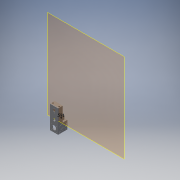
# Autodesk Inventor part: Xendmotorside
Saved by Autodesk Inventor 2016 (Build 200138000, 138)
## iProperties
Created: 2016-05-27
Part Number: Xendmotorside
Material: Generic
Document SubType Name: Modeling
Designer: Scott
Density: 1 g/cm^3
Appearance: Default
Author: Scott
Autodesk Inventor part; units mm, degrees
ref_plane "YZ Plane" through (0, 0, 0) normal (1, 0, 0) x (0, 1, 0)
ref_plane "XZ Plane" through (0, 0, 0) normal (0, 1, 0) x (-1, 0, 0)
ref_plane "XY Plane" through (0, 0, 0) normal (0, 0, 1) x (1, 0, 0)
ref_plane "Work Plane1" through (0, 0, 0) normal (0, 0, 1) x (1, 0, 0)
sketch "Sketch1" plane through (0, 0, 0) normal (0, 0, 1) x (1, 0, 0)
  circle A0 centre (0, 0) radius 6.35 projected
  circle A1 centre (0.5752, -49.1016) radius 4 projected
  line L0 (-12.7, -22.86) -> (12.7, -22.86)
  line L1 (12.7, -22.86) -> (12.7, 22.86)
  line L2 (12.7, 22.86) -> (-12.7, 22.86)
  line L3 (-12.7, 22.86) -> (-12.7, -22.86)
  line L4 (-12.7, -22.86) -> (12.7, 22.86) construction
  line L5 (12.7, -22.86) -> (-12.7, 22.86) construction
  line L6 (12.7, 22.86) -> (-12.7, 22.86)
  line L7 (-12.7, 22.86) -> (-12.7, -66.04)
  line L8 (-12.7, -66.04) -> (12.7, -66.04)
  line L9 (12.7, -66.04) -> (12.7, 22.86)
  point P0 (0, 0)
  dimension "d0" = 25.4
  dimension "d1" = 45.72
  dimension "d2" = 88.9
  constraints: 20 end point, 4 parallel, 2 horizontal, 2 midpoint, 2 perpendicular
  measures "d0" distance of L2.end L1.end
  measures "d1" distance of L1.end L0.end
  measures "d2" distance of L7.end L6.end
extrude "Extrusion1" add sketch "Sketch1" along normal blind 2.54
sketch "Sketch2" plane through (0, 0, 2.54) normal (0, 0, 1) x (1, 0, 0)
  circle A0 centre (0, 0) radius 6.35 projected
  circle A1 centre (0.5752, -49.1016) radius 4 projected
  line L0 (12.7, 22.86) -> (-12.7, 22.86) projected
  line L1 (-12.7, 22.86) -> (-12.7, -66.04) projected
  line L2 (-12.7, -66.04) -> (12.7, -66.04) projected
  line L3 (12.7, -66.04) -> (12.7, 22.86) projected
  circle A2 centre (0, 0) radius 7.62
  line L4 (0, 0) -> (0, -12.7)
  circle A3 centre (0, -12.7) radius 2.54
  line L5 (0, 0) -> (0, 12.7)
  circle A4 centre (0, 12.7) radius 2.54
  circle A5 centre (0.5752, -49.1016) radius 4 projected
  circle A6 centre (0.5752, -49.1016) radius 5
  point P0 (0, 0)
  dimension "d5" = 15.24
  dimension "d6" = 12.7
  dimension "d7" = 5.08
  dimension "d8" = 12.7
  dimension "d9" = 5.08
  dimension "d10" = 10
  constraints: 4 centre point, 4 coincident, 4 end point, 2 vertical
  measures "d5" diameter of A2
  measures "d6" distance of L4.start L4.end
  measures "d7" diameter of A3
  measures "d8" distance of L4.start L5.end
  measures "d9" diameter of A4
  measures "d10" diameter of A6
extrude "Extrusion2" cut sketch "Sketch2" against normal blind 2.54 contours A0 L4 L5 | A0 L5 A2 L4 | L5 L4 A0 | A0 L4 A2 L5 | A3 | A4 | A6
sketch "Sketch3" plane through (0, 0, 0) normal (0, 0, -1) x (-1, 0, 0)
  circle A0 centre (0, 0) radius 7.62 projected
  circle A1 centre (0, 12.7) radius 2.54 projected
  circle A2 centre (0, -12.7) radius 2.54 projected
  circle A3 centre (-0.5752, -49.1016) radius 5 projected
  line L0 (-12.7, 22.86) -> (12.7, 22.86) projected
  line L1 (-12.7, -66.04) -> (-12.7, 22.86) projected
  line L2 (12.7, -66.04) -> (-12.7, -66.04) projected
  line L3 (12.7, 22.86) -> (12.7, -66.04) projected
  line L4 (10.16, 19.05) -> (-10.16, 19.05)
  line L5 (-10.16, 19.05) -> (-10.16, -19.05)
  line L6 (-10.16, -19.05) -> (10.16, -19.05)
  line L7 (10.16, -19.05) -> (10.16, 19.05)
  circle A4 centre (0, 0) radius 7.62 projected
  line L8 (10.16, 19.05) -> (-10.16, -19.05) construction
  line L9 (-10.16, 19.05) -> (10.16, -19.05) construction
  point P0 (0, 0)
  dimension "d13" = 20.32
  dimension "d14" = 38.1
  constraints: 12 end point, 2 midpoint, 2 parallel, 1 horizontal, 1 perpendicular
  measures "d13" distance of L6.end L5.end
  measures "d14" distance of L5.end L4.end
extrude "Extrusion3" add sketch "Sketch3" along normal blind 25.4 contours L0 L3 L2 L1
sketch "Sketch4" plane through (0, 0, 2.54) normal (0, 0, 1) x (1, 0, 0)
  line L0 (-12.7, -66.04) -> (12.7, -66.04) projected
  line L1 (0, -66.04) -> (0, -90.8431)
  line L2 (24.81, -115.6589) -> (-24.81, -115.6589)
  line L3 (-24.81, -115.6589) -> (-24.81, -66.0273)
  line L4 (-24.81, -66.0273) -> (24.81, -66.0273)
  line L5 (24.81, -66.0273) -> (24.81, -115.6589)
  line L6 (24.81, -115.6589) -> (-24.81, -66.0273) construction
  line L7 (-24.81, -115.6589) -> (24.81, -66.0273) construction
  circle A0 centre (0, -90.8431) radius 12.5
  line L8 (0, -90.8431) -> (-15.5, -90.8431)
  line L9 (-15.5, -90.8431) -> (-15.5, -75.3431)
  circle A1 centre (-15.5, -75.3431) radius 2
  circle A2 centre (-15.5, -106.3467) radius 2
  circle A3 centre (15.5, -106.3467) radius 2
  circle A4 centre (15.5, -75.3395) radius 2
  point P0 (0, 0)
  dimension "d17" = 24.8031
  dimension "d18" = 49.62
  dimension "d19" = 49.6316
  dimension "d20" = 25
  dimension "d21" = 15.5
  dimension "d22" = 15.5
  dimension "d23" = 4
  dimension "d24" = 4
  dimension "d25" = 4
  dimension "d26" = 4
  constraints: 18 end point, 5 centre point, 3 midpoint, 3 point on line, 2 coincident, 2 horizontal, 2 parallel, 2 vertical, 1 perpendicular
  measures "d17" distance of L1.start L1.end
  measures "d18" distance of L3.end L4.end
  measures "d19" distance of L2.end L3.end
  measures "d20" diameter of A0
  measures "d21" distance of L8.start L8.end
  measures "d22" distance of L8.end L9.end
  measures "d23" diameter of A1
  measures "d24" diameter of A2
  measures "d25" diameter of A3
  measures "d26" diameter of A4
extrude "Extrusion4" add sketch "Sketch4" against normal blind 5.08
sketch "Sketch5" plane through (0, 0, -2.54) normal (0, 0, -1) x (-1, 0, 0)
  circle A0 centre (0, -90.8431) radius 12.5 projected
  circle A1 centre (-15.5, -75.3395) radius 2 projected
  circle A2 centre (-15.5, -106.3467) radius 2 projected
  circle A3 centre (15.5, -106.3467) radius 2 projected
  circle A4 centre (15.5, -75.3431) radius 2 projected
  line L0 (-12.7, -66.0273) -> (-12.7, 22.86) projected
  line L1 (-12.7, 22.86) -> (12.7, 22.86) projected
  line L2 (12.7, 22.86) -> (12.7, -66.0273) projected
  line L3 (24.81, -66.0273) -> (12.7, -66.0273) projected
  line L4 (24.81, -115.6589) -> (24.81, -66.0273) projected
  line L5 (-24.81, -115.6589) -> (24.81, -115.6589) projected
  line L6 (-24.81, -66.0273) -> (-24.81, -115.6589) projected
  line L7 (-12.7, -66.0273) -> (-24.81, -66.0273) projected
  circle A5 centre (0, 0) radius 7.62 projected
  circle A6 centre (0, 12.7) radius 2.54 projected
  circle A7 centre (0, -12.7) radius 2.54 projected
  circle A8 centre (-0.5752, -49.1016) radius 5 projected
  line L8 (24.81, -66.0273) -> (12.7, -66.0273) projected
  line L9 (-24.81, -115.6589) -> (24.81, -115.6589)
  line L10 (24.81, -115.6589) -> (24.81, -66.0273)
  line L11 (24.81, -66.0273) -> (-24.81, -66.0273)
  line L12 (-24.81, -66.0273) -> (-24.81, -115.6589)
  line L13 (-24.81, -115.6589) -> (24.81, -66.0273) construction
  line L14 (24.81, -115.6589) -> (-24.81, -66.0273) construction
  line L15 (-22, -112.8431) -> (22, -112.8431)
  line L16 (22, -112.8431) -> (22, -68.8431)
  line L17 (22, -68.8431) -> (-22, -68.8431)
  line L18 (-22, -68.8431) -> (-22, -112.8431)
  line L19 (-22, -112.8431) -> (22, -68.8431) construction
  line L20 (22, -112.8431) -> (-22, -68.8431) construction
  point P0 (0, 0)
  dimension "d29" = 44
  dimension "d30" = 44
  constraints: 24 end point, 4 midpoint, 4 parallel, 2 horizontal, 2 perpendicular
  measures "d29" distance of L17.end L16.end
  measures "d30" distance of L16.end L15.end
extrude "Extrusion5" add sketch "Sketch5" along normal blind 50.8 contours L11 L3 L4 L5 L6 L7
sketch "Sketch6" plane through (0, 0, -53.34) normal (0, 0, -1) x (-1, 0, 0)
  line L0 (22, -68.8431) -> (22, -112.8431) projected
  line L1 (22, -112.8431) -> (50.6459, -112.8431)
  line L2 (50.6459, -112.8431) -> (50.6459, -68.8431)
  line L3 (50.6459, -68.8431) -> (22, -68.8431)
  line L4 (22, -68.8431) -> (22, -112.8431)
  point P0 (0, 0)
  constraints: 8 end point, 2 parallel, 1 horizontal, 1 perpendicular
extrude "Extrusion6" cut sketch "Sketch6" against normal blind 50.8
chamfer "Chamfer1" distance 44.45 angle 45 1 edges at (-24.81, -114.251, -53.34)
sketch "Sketch7" plane through (12.7, -66.0273, 2.54) normal (0, 1, 0) x (1, 0, 0)
  line L0 (-25.4, 27.94) -> (-25.4, 0) projected
  line L1 (0, 27.94) -> (-25.4, 27.94) projected
  line L2 (0, 0) -> (0, 27.94) projected
  line L3 (0, 0) -> (12.11, 0) projected
  line L4 (12.11, 0) -> (12.11, 55.88) projected
  line L5 (-37.51, 55.88) -> (12.11, 55.88) projected
  line L6 (-37.51, 0) -> (-37.51, 55.88) projected
  line L7 (-37.51, 0) -> (-25.4, 0) projected
  line L8 (6.055, 0) -> (6.055, 12.7)
  circle A0 centre (6.055, 12.7) radius 4
  circle A1 centre (-31.455, 12.7) radius 4
  line L9 (0, 27.94) -> (12.11, 27.94)
  line L10 (12.11, 0) -> (12.11, 55.88) projected
  line L11 (-25.4, 27.94) -> (-37.51, 27.94)
  line L12 (-37.51, 55.88) -> (-37.51, 5.08) projected
  point P0 (-12.7, 2.54)
  dimension "d38" = 12.7
  dimension "d39" = 8
  dimension "d40" = 8
  constraints: 6 end point, 2 centre point, 2 midpoint, 2 point on line, 1 coincident, 1 vertical
  measures "d38" distance of L8.start L8.end
  measures "d39" diameter of A0
  measures "d40" diameter of A1
extrude "Extrusion7" add sketch "Sketch7" along normal up to surface (88.8873 mm away) contours L0 L7 L6 L11 | L9 L4 L3 L2
sketch "Sketch8" plane through (0, 0, -25.4) normal (0, 0, -1) x (-1, 0, 0)
  line L0 (24.81, -66.0273) -> (-24.81, -66.0273) projected
  line L1 (24.81, -66.0273) -> (24.81, 22.86) projected
  line L2 (24.81, 22.86) -> (-24.81, 22.86) projected
  line L3 (-24.81, -66.0273) -> (-24.81, 22.86) projected
  line L4 (10.16, 19.05) -> (10.16, -19.05) projected
  line L5 (10.16, -19.05) -> (-10.16, -19.05) projected
  line L6 (-10.16, -19.05) -> (-10.16, 19.05) projected
  line L7 (-10.16, 19.05) -> (10.16, 19.05) projected
  circle A0 centre (-0.5752, -49.1016) radius 5 projected
  circle A1 centre (-0.5752, -49.1016) radius 12.7
  point P0 (0, 0)
  dimension "d43" = 25.4
  constraints: 1 centre point, 1 coincident
  measures "d43" diameter of A1
extrude "Extrusion8" add sketch "Sketch8" along normal blind 12.7 contours A1
sketch "Sketch9" plane through (0.5752, -49.1016, -38.1) normal (0, 0, -1) x (-1, 0, 0)
  circle A0 centre (0, 0) radius 12.7 projected
  line L0 (25.3852, -16.9257) -> (-24.2348, -16.9257) projected
  line L1 (25.3852, -16.9257) -> (25.3852, 71.9616) projected
  line L2 (25.3852, 71.9616) -> (-24.2348, 71.9616) projected
  line L3 (-24.2348, -16.9257) -> (-24.2348, 71.9616) projected
  line L4 (10.7352, 68.1516) -> (10.7352, 30.0516) projected
  line L5 (10.7352, 30.0516) -> (-9.5848, 30.0516) projected
  line L6 (-9.5848, 30.0516) -> (-9.5848, 68.1516) projected
  line L7 (-9.5848, 68.1516) -> (10.7352, 68.1516) projected
  line L8 (-12.7, 0) -> (-12.7, -16.9257)
  line L9 (25.3852, -16.9257) -> (-24.2348, -16.9257) projected
  circle A1 centre (0, 0) radius 12.7 projected
  line L10 (12.7, 0) -> (12.7, -16.9257)
  line L11 (12.7, -16.9257) -> (-12.7, -16.9257)
  point P0 (0.5752, 49.1016)
  constraints: 6 end point, 2 perpendicular, 2 point on circle, 2 point on line, 1 collinear, 1 horizontal alignment, 1 vertical, 1 other
extrude "Extrusion9" add sketch "Sketch9" against normal up to surface (12.7 mm away) contours L10 L0 L8 A0
sketch "Sketch10" plane through (0, 0, -38.1) normal (0, 0, -1) x (-1, 0, 0)
  circle A0 centre (-0.5752, -49.1016) radius 5 projected
  circle A1 centre (-0.5752, -49.1016) radius 7.5
  point P0 (0, 0)
  dimension "d48" = 15
  constraints: 1 centre point, 1 coincident
  measures "d48" diameter of A1
sketch "Sketch11" plane through (0, 0, 2.54) normal (0, 0, 1) x (1, 0, 0)
  circle A0 centre (0.5752, -49.1016) radius 5 projected
  circle A1 centre (0.5752, -49.1016) radius 7.5
  point P0 (0, 0)
  dimension "d49" = 15
  constraints: 1 centre point, 1 coincident
  measures "d49" diameter of A1
extrude "Extrusion10" cut sketch "Sketch11" against normal blind 24
sketch "Sketch12" plane through (0, 0, -38.1) normal (0, 0, -1) x (-1, 0, 0)
  circle A0 centre (-0.5752, -49.1016) radius 5 projected
  arc A1 (12.1248, -49.1016) -> (-13.2752, -49.1016) centre (-0.5752, -49.1016) ccw projected
  line L0 (-13.2752, -49.1016) -> (-13.2752, -66.0273) projected
  line L1 (12.1248, -66.0273) -> (-13.2752, -66.0273) projected
  line L2 (12.1248, -66.0273) -> (12.1248, -49.1016) projected
  point P0 (0, 0)
extrude "Extrusion11" add sketch "Sketch12" along normal blind 8.89
sketch "Sketch13" plane through (0, 0, -46.99) normal (0, 0, -1) x (-1, 0, 0)
  circle A0 centre (-0.5752, -49.1016) radius 5 projected
  arc A1 (12.1248, -49.1016) -> (-13.2752, -49.1016) centre (-0.5752, -49.1016) ccw projected
  line L0 (-13.2752, -49.1016) -> (-13.2752, -66.0273) projected
  line L1 (12.1248, -66.0273) -> (-13.2752, -66.0273) projected
  line L2 (12.1248, -66.0273) -> (12.1248, -49.1016) projected
  circle A2 centre (-0.5752, -49.1016) radius 7.5
  point P0 (0, 0)
  dimension "d54" = 15
  constraints: 1 centre point, 1 coincident
  measures "d54" diameter of A2
extrude "Extrusion12" cut sketch "Sketch13" against normal blind 24 contours A2
sketch "Sketch14" plane through (24.81, -115.6589, 2.54) normal (1, 0, 0) x (0, 0, -1)
  spline S0 degree 2 poles (6.6012, 5.0914) (10.3495, 6.6696) (13.0128, 10.9605) knots 0 0 0 1 1 1
  spline S1 degree 2 poles (13.0128, 10.9605) (14.6897, 14.0677) (14.6897, 14.6102) knots 0 0 0 1 1 1
  line L0 (14.6897, 14.6102) -> (14.2952, 14.6102)
  spline S2 degree 2 poles (14.2952, 14.6102) (13.0128, 14.6102) (8.8206, 7.0642) knots 0 0 0 1 1 1
  line L1 (8.8206, 7.0642) -> (8.722, 7.0642)
  line L2 (8.722, 7.0642) -> (8.722, 7.3108)
  spline S3 degree 2 poles (8.722, 7.3108) (11.3359, 12.7854) (11.3359, 16.583) knots 0 0 0 1 1 1
  spline S4 degree 2 poles (11.3359, 16.583) (11.3359, 18.0133) (9.1165, 23.192) knots 0 0 0 1 1 1
  spline S5 degree 2 poles (9.1165, 23.192) (8.574, 25.3621) (8.574, 26.743) knots 0 0 0 1 1 1
  line L3 (8.574, 26.743) -> (8.574, 28.272)
  spline S6 degree 2 poles (8.574, 28.272) (8.574, 35.67) (12.6183, 45.8793) knots 0 0 0 1 1 1
  line L4 (12.6183, 45.8793) -> (12.8649, 46.9151)
  line L5 (12.8649, 46.9151) -> (13.1608, 46.9151)
  line L6 (13.1608, 46.9151) -> (13.1608, 45.0902)
  spline S7 degree 2 poles (13.1608, 45.0902) (13.2594, 42.0817) (13.654, 42.0817) knots 0 0 0 1 1 1
  spline S8 degree 2 poles (13.654, 42.0817) (17.4517, 43.4133) (20.0656, 43.4133) knots 0 0 0 1 1 1
  spline S9 degree 2 poles (20.0656, 43.4133) (24.9484, 43.4133) (30.9654, 38.7279) knots 0 0 0 1 1 1
  spline S10 degree 2 poles (30.9654, 38.7279) (37.0812, 31.6257) (38.9554, 22.3042) knots 0 0 0 1 1 1
  spline S11 degree 2 poles (38.9554, 22.3042) (39.4486, 19.4929) (39.4486, 14.7582) knots 0 0 0 1 1 1
  line L7 (39.4486, 14.7582) -> (39.4486, 13.969)
  spline S12 degree 2 poles (39.4486, 13.969) (41.8159, 7.5574) (46.8466, 5.0914) knots 0 0 0 1 1 1
  spline S13 degree 2 poles (46.8466, 5.0914) (47.2412, 5.0914) (47.2412, 4.8448) knots 0 0 0 1 1 1
  line L8 (47.2412, 4.8448) -> (46.452, 4.5982)
  line L9 (46.452, 4.5982) -> (46.3534, 4.5982)
  spline S14 degree 2 poles (46.3534, 4.5982) (44.4299, 4.5982) (39.5472, 9.7768) knots 0 0 0 1 1 1
  line L10 (39.5472, 9.7768) -> (39.5472, 9.6782)
  line L11 (39.5472, 9.6782) -> (39.6952, 7.5574)
  line L12 (39.6952, 7.5574) -> (39.6952, 7.3108)
  line L13 (39.6952, 7.3108) -> (39.4486, 7.3108)
  spline S15 degree 2 poles (39.4486, 7.3108) (38.1169, 12.7854) (35.6509, 14.6102) knots 0 0 0 1 1 1
  spline S16 degree 2 poles (35.6509, 14.6102) (35.6509, 14.8568) (34.3686, 14.8568) knots 0 0 0 1 1 1
  line L14 (34.3686, 14.8568) -> (31.3107, 14.8568)
  line L15 (31.3107, 14.8568) -> (31.3107, 11.7496)
  spline S17 degree 2 poles (31.3107, 11.7496) (31.3107, 11.3057) (33.2342, 10.9605) knots 0 0 0 1 1 1
  line L16 (33.2342, 10.9605) -> (33.2342, 10.7139)
  line L17 (33.2342, 10.7139) -> (26.0334, 10.7139)
  line L18 (26.0334, 10.7139) -> (26.0334, 10.9605)
  spline S18 degree 2 poles (26.0334, 10.9605) (26.6746, 10.9605) (27.3157, 12.1442) knots 0 0 0 1 1 1
  line L19 (27.3157, 12.1442) -> (27.3157, 14.8568)
  line L20 (27.3157, 14.8568) -> (21.5946, 14.8568)
  line L21 (21.5946, 14.8568) -> (21.348, 15.1527)
  line L22 (21.348, 15.1527) -> (21.5946, 16.2871)
  spline S19 degree 2 poles (21.5946, 16.2871) (21.2493, 17.8654) (20.0656, 17.8654) knots 0 0 0 1 1 1
  spline S20 degree 2 poles (20.0656, 17.8654) (18.3887, 17.8654) (17.6983, 14.3636) knots 0 0 0 1 1 1
  spline S21 degree 2 poles (17.6983, 14.3636) (16.12, 11.6017) (10.9414, 6.5217) knots 0 0 0 1 1 1
  spline S22 degree 2 poles (10.9414, 6.5217) (8.5247, 4.7461) (7.5383, 4.7461) knots 0 0 0 1 1 1
  line L23 (7.5383, 4.7461) -> (7.3903, 4.7461)
  spline S23 degree 2 poles (7.3903, 4.7461) (6.6012, 4.8448) (6.6012, 5.0914) knots 0 0 0 1 1 1
  line L24 (17.6983, 20.6273) -> (27.3157, 20.6273)
  spline S24 degree 2 poles (27.3157, 20.6273) (27.3157, 22.4522) (25.0963, 23.0933) knots 0 0 0 1 1 1
  spline S25 degree 2 poles (25.0963, 23.0933) (24.7511, 23.0933) (24.7511, 23.3399) knots 0 0 0 1 1 1
  line L25 (24.7511, 23.3399) -> (24.7511, 23.4879)
  line L26 (24.7511, 23.4879) -> (33.9247, 23.4879)
  spline S26 degree 2 poles (33.9247, 23.4879) (33.7274, 22.9947) (31.7053, 22.3042) knots 0 0 0 1 1 1
  line L27 (31.7053, 22.3042) -> (31.3107, 20.6273)
  line L28 (31.3107, 20.6273) -> (34.6152, 20.6273)
  spline S27 degree 2 poles (34.6152, 20.6273) (34.2206, 23.8331) (33.3328, 26.3485) knots 0 0 0 1 1 1
  spline S28 degree 2 poles (33.3328, 26.3485) (32.2478, 28.9131) (29.9297, 31.2805) knots 0 0 0 1 1 1
  line L29 (29.9297, 31.2805) -> (29.9297, 31.4285)
  line L30 (29.9297, 31.4285) -> (30.5709, 31.4285)
  spline S29 degree 2 poles (30.5709, 31.4285) (32.7903, 31.0832) (36.3414, 22.6988) knots 0 0 0 1 1 1
  line L31 (36.3414, 22.6988) -> (36.9825, 20.6273)
  spline S30 degree 2 poles (36.9825, 20.6273) (37.821, 20.6273) (38.0183, 21.7617) knots 0 0 0 1 1 1
  spline S31 degree 2 poles (38.0183, 21.7617) (35.7495, 30.0968) (30.3243, 33.8945) knots 0 0 0 1 1 1
  spline S32 degree 2 poles (30.3243, 33.8945) (26.132, 37.1496) (20.7068, 37.1496) knots 0 0 0 1 1 1
  spline S33 degree 2 poles (20.7068, 37.1496) (14.2952, 37.1496) (11.4346, 32.0696) knots 0 0 0 1 1 1
  spline S34 degree 2 poles (11.4346, 32.0696) (10.7934, 30.2448) (10.7934, 28.4199) knots 0 0 0 1 1 1
  spline S35 degree 2 poles (10.7934, 28.4199) (10.7934, 22.9947) (13.1608, 21.5151) knots 0 0 0 1 1 1
  spline S36 degree 2 poles (13.1608, 21.5151) (14.5911, 20.6273) (17.6983, 20.6273) knots 0 0 0 1 1 1
  point P0 (2.54, 115.6589)
  point P1 (6.6012, 7.5081)
  constraints: 1 other
extrude "Extrusion13" add sketch "Sketch14" along normal blind 1.27
sketch "Sketch15" plane through (24.81, -115.6589, 2.54) normal (1, 0, 0) x (0, 0, -1)
  spline S0 degree 2 poles (44.1908, 6.1802) (45.1279, 6.5747) (45.7937, 7.6474) knots 0 0 0 1 1 1
  spline S1 degree 2 poles (45.7937, 7.6474) (46.2129, 8.4242) (46.2129, 8.5599) knots 0 0 0 1 1 1
  line L0 (46.2129, 8.5599) -> (46.1143, 8.5599)
  spline S2 degree 2 poles (46.1143, 8.5599) (45.7937, 8.5599) (44.7457, 6.6734) knots 0 0 0 1 1 1
  line L1 (44.7457, 6.6734) -> (44.721, 6.6734)
  line L2 (44.721, 6.6734) -> (44.721, 6.735)
  spline S3 degree 2 poles (44.721, 6.735) (45.3745, 8.1036) (45.3745, 9.0531) knots 0 0 0 1 1 1
  spline S4 degree 2 poles (45.3745, 9.0531) (45.3745, 9.4106) (44.8196, 10.7053) knots 0 0 0 1 1 1
  spline S5 degree 2 poles (44.8196, 10.7053) (44.684, 11.2478) (44.684, 11.5931) knots 0 0 0 1 1 1
  line L3 (44.684, 11.5931) -> (44.684, 11.9753)
  spline S6 degree 2 poles (44.684, 11.9753) (44.684, 13.8248) (45.6951, 16.3771) knots 0 0 0 1 1 1
  line L4 (45.6951, 16.3771) -> (45.7567, 16.6361)
  line L5 (45.7567, 16.6361) -> (45.8307, 16.6361)
  line L6 (45.8307, 16.6361) -> (45.8307, 16.1799)
  spline S7 degree 2 poles (45.8307, 16.1799) (45.8554, 15.4277) (45.954, 15.4277) knots 0 0 0 1 1 1
  spline S8 degree 2 poles (45.954, 15.4277) (46.9034, 15.7606) (47.5569, 15.7606) knots 0 0 0 1 1 1
  spline S9 degree 2 poles (47.5569, 15.7606) (48.7776, 15.7606) (50.2819, 14.5893) knots 0 0 0 1 1 1
  spline S10 degree 2 poles (50.2819, 14.5893) (51.8108, 12.8137) (52.2793, 10.4834) knots 0 0 0 1 1 1
  spline S11 degree 2 poles (52.2793, 10.4834) (52.4026, 9.7805) (52.4026, 8.5969) knots 0 0 0 1 1 1
  line L7 (52.4026, 8.5969) -> (52.4026, 8.3996)
  spline S12 degree 2 poles (52.4026, 8.3996) (52.9945, 6.7967) (54.2522, 6.1802) knots 0 0 0 1 1 1
  spline S13 degree 2 poles (54.2522, 6.1802) (54.3508, 6.1802) (54.3508, 6.1185) knots 0 0 0 1 1 1
  line L8 (54.3508, 6.1185) -> (54.1535, 6.0569)
  line L9 (54.1535, 6.0569) -> (54.1289, 6.0569)
  spline S14 degree 2 poles (54.1289, 6.0569) (53.648, 6.0569) (52.4273, 7.3515) knots 0 0 0 1 1 1
  line L10 (52.4273, 7.3515) -> (52.4273, 7.3269)
  line L11 (52.4273, 7.3269) -> (52.4643, 6.7967)
  line L12 (52.4643, 6.7967) -> (52.4643, 6.735)
  line L13 (52.4643, 6.735) -> (52.4026, 6.735)
  spline S15 degree 2 poles (52.4026, 6.735) (52.0697, 8.1036) (51.4532, 8.5599) knots 0 0 0 1 1 1
  spline S16 degree 2 poles (51.4532, 8.5599) (51.4532, 8.6215) (51.1326, 8.6215) knots 0 0 0 1 1 1
  line L14 (51.1326, 8.6215) -> (50.3682, 8.6215)
  line L15 (50.3682, 8.6215) -> (50.3682, 7.8447)
  spline S17 degree 2 poles (50.3682, 7.8447) (50.3682, 7.7337) (50.8491, 7.6474) knots 0 0 0 1 1 1
  line L16 (50.8491, 7.6474) -> (50.8491, 7.5858)
  line L17 (50.8491, 7.5858) -> (49.0489, 7.5858)
  line L18 (49.0489, 7.5858) -> (49.0489, 7.6474)
  spline S18 degree 2 poles (49.0489, 7.6474) (49.2092, 7.6474) (49.3694, 7.9434) knots 0 0 0 1 1 1
  line L19 (49.3694, 7.9434) -> (49.3694, 8.6215)
  line L20 (49.3694, 8.6215) -> (47.9392, 8.6215)
  line L21 (47.9392, 8.6215) -> (47.8775, 8.6955)
  line L22 (47.8775, 8.6955) -> (47.9392, 8.9791)
  spline S19 degree 2 poles (47.9392, 8.9791) (47.8528, 9.3736) (47.5569, 9.3736) knots 0 0 0 1 1 1
  spline S20 degree 2 poles (47.5569, 9.3736) (47.1377, 9.3736) (46.9651, 8.4982) knots 0 0 0 1 1 1
  spline S21 degree 2 poles (46.9651, 8.4982) (46.5705, 7.8077) (45.2759, 6.5377) knots 0 0 0 1 1 1
  spline S22 degree 2 poles (45.2759, 6.5377) (44.6717, 6.0938) (44.4251, 6.0938) knots 0 0 0 1 1 1
  line L23 (44.4251, 6.0938) -> (44.3881, 6.0938)
  spline S23 degree 2 poles (44.3881, 6.0938) (44.1908, 6.1185) (44.1908, 6.1802) knots 0 0 0 1 1 1
  line L24 (46.9651, 10.0641) -> (49.3694, 10.0641)
  spline S24 degree 2 poles (49.3694, 10.0641) (49.3694, 10.5203) (48.8146, 10.6806) knots 0 0 0 1 1 1
  spline S25 degree 2 poles (48.8146, 10.6806) (48.7283, 10.6806) (48.7283, 10.7423) knots 0 0 0 1 1 1
  line L25 (48.7283, 10.7423) -> (48.7283, 10.7793)
  line L26 (48.7283, 10.7793) -> (51.0217, 10.7793)
  spline S26 degree 2 poles (51.0217, 10.7793) (50.9724, 10.656) (50.4668, 10.4834) knots 0 0 0 1 1 1
  line L27 (50.4668, 10.4834) -> (50.3682, 10.0641)
  line L28 (50.3682, 10.0641) -> (51.1943, 10.0641)
  spline S27 degree 2 poles (51.1943, 10.0641) (51.0957, 10.8656) (50.8737, 11.4944) knots 0 0 0 1 1 1
  spline S28 degree 2 poles (50.8737, 11.4944) (50.6025, 12.1356) (50.0229, 12.7274) knots 0 0 0 1 1 1
  line L29 (50.0229, 12.7274) -> (50.0229, 12.7644)
  line L30 (50.0229, 12.7644) -> (50.1832, 12.7644)
  spline S29 degree 2 poles (50.1832, 12.7644) (50.7381, 12.6781) (51.6259, 10.582) knots 0 0 0 1 1 1
  line L31 (51.6259, 10.582) -> (51.7861, 10.0641)
  spline S30 degree 2 poles (51.7861, 10.0641) (51.9958, 10.0641) (52.0451, 10.3477) knots 0 0 0 1 1 1
  spline S31 degree 2 poles (52.0451, 10.3477) (51.4779, 12.4315) (50.1216, 13.3809) knots 0 0 0 1 1 1
  spline S32 degree 2 poles (50.1216, 13.3809) (49.0735, 14.1947) (47.7172, 14.1947) knots 0 0 0 1 1 1
  spline S33 degree 2 poles (47.7172, 14.1947) (46.1143, 14.1947) (45.3992, 12.9247) knots 0 0 0 1 1 1
  spline S34 degree 2 poles (45.3992, 12.9247) (45.2389, 12.4685) (45.2389, 12.0123) knots 0 0 0 1 1 1
  spline S35 degree 2 poles (45.2389, 12.0123) (45.2389, 10.656) (45.8307, 10.2861) knots 0 0 0 1 1 1
  spline S36 degree 2 poles (45.8307, 10.2861) (46.1883, 10.0641) (46.9651, 10.0641) knots 0 0 0 1 1 1
  line L32 (45.0169, 21.8764) -> (45.806, 21.0502)
  spline S37 degree 2 poles (45.806, 21.0502) (45.806, 21.1859) (45.8677, 21.1859) knots 0 0 0 1 1 1
  line L33 (45.8677, 21.1859) -> (45.9417, 21.1859)
  spline S38 degree 2 poles (45.9417, 21.1859) (45.9787, 21.1859) (46.0526, 20.9393) knots 0 0 0 1 1 1
  line L34 (46.0526, 20.9393) -> (46.1636, 20.7913)
  line L35 (46.1636, 20.7913) -> (46.3856, 20.8283)
  spline S39 degree 2 poles (46.3856, 20.8283) (47.187, 20.8283) (48.2597, 19.8049) knots 0 0 0 1 1 1
  spline S40 degree 2 poles (48.2597, 19.8049) (49.0119, 19.509) (49.1105, 19.509) knots 0 0 0 1 1 1
  line L36 (49.1105, 19.509) -> (51.4409, 19.509)
  spline S41 degree 2 poles (51.4409, 19.509) (51.7122, 19.509) (51.9711, 19.6939) knots 0 0 0 1 1 1
  spline S42 degree 2 poles (51.9711, 19.6939) (52.1067, 19.6939) (52.1067, 19.9405) knots 0 0 0 1 1 1
  line L37 (52.1067, 19.9405) -> (52.3163, 20.3844)
  line L38 (52.3163, 20.3844) -> (52.378, 20.3844)
  line L39 (52.378, 20.3844) -> (52.2793, 19.3117)
  spline S43 degree 2 poles (52.2793, 19.3117) (52.2793, 18.4733) (52.4273, 17.4622) knots 0 0 0 1 1 1
  line L40 (52.4273, 17.4622) -> (52.378, 17.4622)
  spline S44 degree 2 poles (52.378, 17.4622) (52.2177, 18.017) (52.0697, 18.1897) knots 0 0 0 1 1 1
  spline S45 degree 2 poles (52.0697, 18.1897) (52.0697, 18.4239) (51.8355, 18.4239) knots 0 0 0 1 1 1
  spline S46 degree 2 poles (51.8355, 18.4239) (51.5395, 18.5226) (50.0969, 18.6212) knots 0 0 0 1 1 1
  spline S47 degree 2 poles (50.0969, 18.6212) (49.3325, 18.6212) (48.6666, 18.2636) knots 0 0 0 1 1 1
  spline S48 degree 2 poles (48.6666, 18.2636) (46.4595, 17.4129) (46.3609, 17.2526) knots 0 0 0 1 1 1
  line L41 (46.3609, 17.2526) -> (46.3609, 17.1663)
  spline S49 degree 2 poles (46.3609, 17.1663) (46.3609, 16.9443) (46.4842, 16.3155) knots 0 0 0 1 1 1
  line L42 (46.4842, 16.3155) -> (46.4472, 16.3155)
  spline S50 degree 2 poles (46.4472, 16.3155) (46.102, 17.0306) (46.0526, 17.0306) knots 0 0 0 1 1 1
  spline S51 degree 2 poles (46.0526, 17.0306) (45.991, 16.8087) (45.9417, 16.8087) knots 0 0 0 1 1 1
  line L43 (45.9417, 16.8087) -> (45.8677, 16.8087)
  line L44 (45.8677, 16.8087) -> (45.806, 16.858)
  line L45 (45.806, 16.858) -> (45.806, 17.5855)
  line L46 (45.806, 17.5855) -> (45.6088, 18.0664)
  spline S52 degree 2 poles (45.6088, 18.0664) (45.806, 18.1403) (45.806, 18.1897) knots 0 0 0 1 1 1
  line L47 (45.806, 18.1897) -> (45.806, 18.5472)
  line L48 (45.806, 18.5472) -> (45.8677, 18.5966)
  line L49 (45.8677, 18.5966) -> (45.9417, 18.5966)
  spline S53 degree 2 poles (45.9417, 18.5966) (45.991, 18.5966) (46.0526, 18.2636) knots 0 0 0 1 1 1
  spline S54 degree 2 poles (46.0526, 18.2636) (47.1377, 18.7938) (48.0871, 19.398) knots 0 0 0 1 1 1
  spline S55 degree 2 poles (48.0871, 19.398) (48.0871, 19.6323) (47.4336, 19.8049) knots 0 0 0 1 1 1
  spline S56 degree 2 poles (47.4336, 19.8049) (46.7555, 20.1132) (46.5828, 20.1132) knots 0 0 0 1 1 1
  line L50 (46.5828, 20.1132) -> (46.4842, 20.1132)
  spline S57 degree 2 poles (46.4842, 20.1132) (46.3239, 20.0269) (46.3239, 19.7802) knots 0 0 0 1 1 1
  line L51 (46.3239, 19.7802) -> (46.4102, 19.1514)
  line L52 (46.4102, 19.1514) -> (46.1143, 19.62)
  spline S58 degree 2 poles (46.1143, 19.62) (46.0403, 19.62) (46.0033, 19.7186) knots 0 0 0 1 1 1
  spline S59 degree 2 poles (46.0033, 19.7186) (45.806, 19.7186) (45.806, 19.7802) knots 0 0 0 1 1 1
  line L53 (45.806, 19.7802) -> (45.806, 19.9775)
  line L54 (45.806, 19.9775) -> (45.7567, 19.9775)
  line L55 (45.7567, 19.9775) -> (45.7567, 20.0515)
  spline S60 degree 2 poles (45.7567, 20.0515) (45.7567, 20.1748) (45.0169, 21.8517) knots 0 0 0 1 1 1
  line L56 (45.0169, 21.8517) -> (45.0169, 21.8764)
  spline S61 degree 2 poles (45.7937, 26.3029) (45.8307, 26.5371) (45.88, 26.5371) knots 0 0 0 1 1 1
  line L57 (45.88, 26.5371) -> (45.991, 26.5371)
  line L58 (45.991, 26.5371) -> (46.0403, 26.4755)
  line L59 (46.0403, 26.4755) -> (46.0403, 26.2166)
  spline S62 degree 2 poles (46.0403, 26.2166) (46.0403, 25.8343) (46.6198, 25.785) knots 0 0 0 1 1 1
  line L60 (46.6198, 25.785) -> (47.6926, 25.7603)
  line L61 (47.6926, 25.7603) -> (52.452, 25.7603)
  line L62 (52.452, 25.7603) -> (52.5013, 25.711)
  line L63 (52.5013, 25.711) -> (52.5013, 25.6617)
  spline S63 degree 2 poles (52.5013, 25.6617) (52.3657, 25.5014) (51.7368, 25.1315) knots 0 0 0 1 1 1
  line L64 (51.7368, 25.1315) -> (51.7368, 25.0945)
  spline S64 degree 2 poles (51.7368, 25.0945) (52.3163, 24.7493) (52.7479, 24.0588) knots 0 0 0 1 1 1
  line L65 (52.7479, 24.0588) -> (53.1918, 23.5533)
  line L66 (53.1918, 23.5533) -> (53.1918, 23.5286)
  line L67 (53.1918, 23.5286) -> (53.0068, 23.6642)
  line L68 (53.0068, 23.6642) -> (53.3274, 23.134)
  spline S65 degree 2 poles (53.3274, 23.134) (51.8478, 24.5767) (51.2806, 24.7739) knots 0 0 0 1 1 1
  line L69 (51.2806, 24.7739) -> (51.2806, 24.8109)
  line L70 (51.2806, 24.8109) -> (47.7665, 22.4682)
  line L71 (47.7665, 22.4682) -> (50.8367, 22.4436)
  line L72 (50.8367, 22.4436) -> (51.3546, 22.4436)
  spline S66 degree 2 poles (51.3546, 22.4436) (51.7738, 22.4436) (52.0081, 22.6532) knots 0 0 0 1 1 1
  line L73 (52.0081, 22.6532) -> (52.3163, 23.097)
  line L74 (52.3163, 23.097) -> (52.341, 23.097)
  line L75 (52.341, 23.097) -> (52.341, 22.9121)
  line L76 (52.341, 22.9121) -> (52.3903, 22.8381)
  line L77 (52.3903, 22.8381) -> (52.3903, 21.0872)
  line L78 (52.3903, 21.0872) -> (52.341, 21.0379)
  line L79 (52.341, 21.0379) -> (52.2424, 21.0379)
  line L80 (52.2424, 21.0379) -> (52.1807, 21.0872)
  line L81 (52.1807, 21.0872) -> (52.1807, 21.2969)
  spline S67 degree 2 poles (52.1807, 21.2969) (52.1807, 21.7777) (51.3546, 21.7777) knots 0 0 0 1 1 1
  line L82 (51.3546, 21.7777) -> (46.9158, 21.7777)
  spline S68 degree 2 poles (46.9158, 21.7777) (47.0267, 21.4078) (47.9268, 20.4707) knots 0 0 0 1 1 1
  line L83 (47.9268, 20.4707) -> (48.0378, 20.3474)
  line L84 (48.0378, 20.3474) -> (48.0378, 20.3104)
  spline S69 degree 2 poles (48.0378, 20.3104) (47.0637, 21.1242) (46.4102, 21.4325) knots 0 0 0 1 1 1
  line L85 (46.4102, 21.4325) -> (46.4102, 21.4818)
  line L86 (46.4102, 21.4818) -> (46.5212, 21.6174)
  line L87 (46.5212, 21.6174) -> (46.5212, 21.6421)
  spline S70 degree 2 poles (46.5212, 21.6421) (46.0157, 21.2969) (46.0157, 20.742) knots 0 0 0 1 1 1
  line L88 (46.0157, 20.742) -> (45.88, 20.742)
  line L89 (45.88, 20.742) -> (45.8307, 20.7913)
  line L90 (45.8307, 20.7913) -> (45.8307, 22.1476)
  line L91 (45.8307, 22.1476) -> (45.991, 22.3079)
  spline S71 degree 2 poles (45.991, 22.3079) (45.9293, 22.3202) (45.88, 22.4436) knots 0 0 0 1 1 1
  spline S72 degree 2 poles (45.88, 22.4436) (46.1266, 23.3683) (47.3103, 24.6753) knots 0 0 0 1 1 1
  spline S73 degree 2 poles (47.3103, 24.6753) (47.372, 24.6753) (47.8159, 25.0945) knots 0 0 0 1 1 1
  line L92 (47.8159, 25.0945) -> (47.8159, 25.1315)
  line L93 (47.8159, 25.1315) -> (46.6568, 25.1315)
  spline S74 degree 2 poles (46.6568, 25.1315) (46.0403, 25.1315) (46.0403, 24.2437) knots 0 0 0 1 1 1
  line L94 (46.0403, 24.2437) -> (45.991, 24.2437)
  line L95 (45.991, 24.2437) -> (45.991, 24.3301)
  spline S75 degree 2 poles (45.991, 24.3301) (45.991, 24.6753) (45.8554, 24.6753) knots 0 0 0 1 1 1
  line L96 (45.8554, 24.6753) -> (45.8307, 24.7)
  line L97 (45.8307, 24.7) -> (45.8307, 26.1919)
  line L98 (45.8307, 26.1919) -> (45.7937, 26.3029)
  line L99 (47.4213, 23.2573) -> (47.4459, 23.2573)
  line L100 (47.4459, 23.2573) -> (50.1339, 25.0205)
  line L101 (50.1339, 25.0205) -> (50.1339, 25.0452)
  line L102 (50.1339, 25.0452) -> (50.0353, 25.0452)
  spline S76 degree 2 poles (50.0353, 25.0452) (48.8269, 25.0452) (47.6679, 23.6396) knots 0 0 0 1 1 1
  line L103 (47.6679, 23.6396) -> (47.4213, 23.2573)
  line L104 (50.5161, 25.3904) -> (50.6888, 25.3904)
  line L105 (50.6888, 25.3904) -> (50.6888, 25.4151)
  line L106 (50.6888, 25.4151) -> (50.5161, 25.4151)
  line L107 (50.5161, 25.4151) -> (50.5161, 25.3904)
  line L108 (44.9553, 27.4372) -> (44.9553, 27.4619)
  line L109 (44.9553, 27.4619) -> (45.7321, 29.2128)
  line L110 (45.7321, 29.2128) -> (45.7321, 29.3854)
  line L111 (45.7321, 29.3854) -> (45.7567, 29.3854)
  line L112 (45.7567, 29.3854) -> (45.7814, 29.3607)
  line L113 (45.7814, 29.3607) -> (45.806, 29.3607)
  line L114 (45.806, 29.3607) -> (45.7814, 29.9772)
  line L115 (45.7814, 29.9772) -> (45.7814, 31.1116)
  spline S77 degree 2 poles (45.7814, 31.1116) (45.8184, 31.1856) (46.5459, 31.6541) knots 0 0 0 1 1 1
  line L116 (46.5459, 31.6541) -> (46.5705, 31.6541)
  line L117 (46.5705, 31.6541) -> (46.5705, 31.6171)
  spline S78 degree 2 poles (46.5705, 31.6171) (46.2623, 31.1239) (46.2623, 30.976) knots 0 0 0 1 1 1
  spline S79 degree 2 poles (46.2623, 30.976) (46.2623, 30.8034) (46.4595, 30.8034) knots 0 0 0 1 1 1
  line L118 (46.4595, 30.8034) -> (51.8108, 30.828)
  spline S80 degree 2 poles (51.8108, 30.828) (52.0944, 30.828) (52.1684, 31.2842) knots 0 0 0 1 1 1
  line L119 (52.1684, 31.2842) -> (52.23, 31.2842)
  spline S81 degree 2 poles (52.23, 31.2842) (52.341, 31.2472) (52.341, 31.1609) knots 0 0 0 1 1 1
  line L120 (52.341, 31.1609) -> (52.3657, 31.1609)
  line L121 (52.3657, 31.1609) -> (52.9082, 31.6788)
  line L122 (52.9082, 31.6788) -> (52.9082, 31.6541)
  spline S82 degree 2 poles (52.9082, 31.6541) (52.341, 30.9883) (52.341, 30.3718) knots 0 0 0 1 1 1
  line L123 (52.341, 30.3718) -> (52.341, 29.0525)
  line L124 (52.341, 29.0525) -> (52.3163, 29.0155)
  line L125 (52.3163, 29.0155) -> (52.3163, 28.9908)
  spline S83 degree 2 poles (52.3163, 28.9908) (52.156, 28.9908) (52.156, 29.2991) knots 0 0 0 1 1 1
  spline S84 degree 2 poles (52.156, 29.2991) (51.9834, 29.7553) (51.7122, 29.7553) knots 0 0 0 1 1 1
  line L126 (51.7122, 29.7553) -> (50.2202, 29.7553)
  line L127 (50.2202, 29.7553) -> (50.2202, 27.6592)
  line L128 (50.2202, 27.6592) -> (50.2572, 27.6592)
  spline S85 degree 2 poles (50.2572, 27.6592) (51.9218, 28.1031) (51.9218, 28.4606) knots 0 0 0 1 1 1
  line L129 (51.9218, 28.4606) -> (51.9464, 28.4236)
  line L130 (51.9464, 28.4236) -> (52.0081, 28.4236)
  line L131 (52.0081, 28.4236) -> (52.3163, 28.7689)
  line L132 (52.3163, 28.7689) -> (52.341, 28.7689)
  line L133 (52.341, 28.7689) -> (52.341, 28.5963)
  line L134 (52.341, 28.5963) -> (52.3657, 28.4606)
  line L135 (52.3657, 28.4606) -> (52.3903, 28.4606)
  spline S86 degree 2 poles (52.3903, 28.4606) (53.6973, 29.2498) (53.8946, 29.2498) knots 0 0 0 1 1 1
  spline S87 degree 2 poles (53.8946, 29.2498) (52.5383, 27.8811) (52.5383, 27.7702) knots 0 0 0 1 1 1
  line L136 (52.5383, 27.7702) -> (52.452, 27.5729)
  line L137 (52.452, 27.5729) -> (52.6493, 25.97)
  line L138 (52.6493, 25.97) -> (52.5999, 25.97)
  line L139 (52.5999, 25.97) -> (52.3657, 26.6358)
  line L140 (52.3657, 26.6358) -> (52.341, 26.6358)
  line L141 (52.341, 26.6358) -> (52.341, 25.2548)
  line L142 (52.341, 25.2548) -> (52.3163, 25.2548)
  spline S88 degree 2 poles (52.3163, 25.2548) (52.1191, 25.2548) (52.0574, 25.711) knots 0 0 0 1 1 1
  spline S89 degree 2 poles (52.0574, 25.711) (51.6752, 26.1919) (50.8984, 26.7344) knots 0 0 0 1 1 1
  spline S90 degree 2 poles (50.8984, 26.7344) (50.4422, 26.6111) (50.0846, 26.6111) knots 0 0 0 1 1 1
  line L143 (50.0846, 26.6111) -> (49.6777, 26.6111)
  spline S91 degree 2 poles (49.6777, 26.6111) (47.9638, 26.6111) (46.5459, 28.1894) knots 0 0 0 1 1 1
  spline S92 degree 2 poles (46.5459, 28.1894) (46.1513, 28.7936) (46.1513, 28.8799) knots 0 0 0 1 1 1
  line L144 (46.1513, 28.8799) -> (46.1143, 28.8799)
  spline S93 degree 2 poles (46.1143, 28.8799) (46.1143, 28.6086) (45.2142, 27.6838) knots 0 0 0 1 1 1
  spline S94 degree 2 poles (45.2142, 27.6838) (45.0416, 27.4372) (44.9553, 27.4372) knots 0 0 0 1 1 1
  line L145 (49.8257, 27.9181) -> (49.8257, 29.7553)
  line L146 (49.8257, 29.7553) -> (47.9885, 29.7553)
  line L147 (47.9885, 29.7553) -> (47.9885, 29.2498)
  line L148 (47.9885, 29.2498) -> (49.8257, 27.9181)
  line L149 (49.2585, 27.5729) -> (49.653, 27.5729)
  spline S95 degree 2 poles (49.653, 27.5729) (49.6284, 27.6345) (49.2585, 27.8565) knots 0 0 0 1 1 1
  line L150 (49.2585, 27.8565) -> (49.2955, 27.8811)
  line L151 (49.2955, 27.8811) -> (48.1858, 28.6456)
  line L152 (48.1858, 28.6456) -> (48.1611, 28.6456)
  line L153 (48.1611, 28.6456) -> (48.1611, 28.6209)
  spline S96 degree 2 poles (48.1611, 28.6209) (48.6173, 28.0661) (49.2338, 27.8811) knots 0 0 0 1 1 1
  line L154 (49.2338, 27.8811) -> (49.2338, 27.8565)
  line L155 (49.2338, 27.8565) -> (49.1722, 27.8565)
  spline S97 degree 2 poles (49.1722, 27.8565) (47.9392, 28.214) (47.5693, 28.4606) knots 0 0 0 1 1 1
  line L156 (47.5693, 28.4606) -> (47.5323, 28.473)
  line L157 (47.5323, 28.473) -> (47.5323, 28.51)
  line L158 (47.5323, 28.51) -> (47.5693, 29.1018)
  spline S98 degree 2 poles (47.5693, 29.1018) (46.6938, 29.7553) (46.5705, 29.7553) knots 0 0 0 1 1 1
  line L159 (46.5705, 29.7553) -> (46.3239, 29.7553)
  spline S99 degree 2 poles (46.3239, 29.7553) (46.3239, 29.0402) (46.9158, 28.5346) knots 0 0 0 1 1 1
  spline S100 degree 2 poles (46.9158, 28.5346) (48.0255, 27.5729) (49.2585, 27.5729) knots 0 0 0 1 1 1
  spline S101 degree 2 poles (51.8848, 26.5618) (52.156, 26.6111) (52.156, 27.0427) knots 0 0 0 1 1 1
  line L160 (52.156, 27.0427) -> (52.156, 27.092)
  line L161 (52.156, 27.092) -> (52.0081, 27.092)
  spline S102 degree 2 poles (52.0081, 27.092) (51.8108, 27.092) (51.2929, 26.8947) knots 0 0 0 1 1 1
  line L162 (51.2929, 26.8947) -> (51.2929, 26.8701)
  spline S103 degree 2 poles (51.2929, 26.8701) (51.6752, 26.5618) (51.8848, 26.5618) knots 0 0 0 1 1 1
  line L163 (47.5693, 29.5334) -> (47.5939, 29.5334)
  line L164 (47.5939, 29.5334) -> (47.5939, 29.7183)
  line L165 (47.5939, 29.7183) -> (47.5323, 29.7183)
  line L166 (47.5323, 29.7183) -> (47.5323, 29.7553)
  line L167 (47.5323, 29.7553) -> (47.3103, 29.7183)
  line L168 (47.3103, 29.7183) -> (47.5693, 29.5334)
  line L169 (45.6951, 32.9735) -> (45.6951, 33.0351)
  spline S104 degree 2 poles (45.6951, 33.0351) (46.9034, 33.8736) (47.8035, 34.4161) knots 0 0 0 1 1 1
  line L170 (47.8035, 34.4161) -> (47.8035, 34.5024)
  spline S105 degree 2 poles (47.8035, 34.5024) (47.0021, 35.1189) (45.8677, 35.7601) knots 0 0 0 1 1 1
  line L171 (45.8677, 35.7601) -> (45.8307, 35.7847)
  line L172 (45.8307, 35.7847) -> (45.8307, 35.8217)
  line L173 (45.8307, 35.8217) -> (45.8677, 36.6355)
  line L174 (45.8677, 36.6355) -> (45.8307, 37.5602)
  line L175 (45.8307, 37.5602) -> (45.8924, 37.5602)
  line L176 (45.8924, 37.5602) -> (45.8924, 37.5356)
  spline S106 degree 2 poles (45.8924, 37.5356) (45.8924, 37.2273) (46.028, 37.2273) knots 0 0 0 1 1 1
  spline S107 degree 2 poles (46.028, 37.2273) (46.028, 36.6848) (46.5705, 36.6848) knots 0 0 0 1 1 1
  line L177 (46.5705, 36.6848) -> (46.8788, 36.6602)
  line L178 (46.8788, 36.6602) -> (51.3669, 36.6602)
  line L179 (51.3669, 36.6602) -> (51.6259, 36.6355)
  spline S108 degree 2 poles (51.6259, 36.6355) (52.1807, 36.6355) (52.1807, 37.252) knots 0 0 0 1 1 1
  line L180 (52.1807, 37.252) -> (52.3533, 37.252)
  line L181 (52.3533, 37.252) -> (52.3533, 34.9463)
  line L182 (52.3533, 34.9463) -> (52.3287, 34.9463)
  line L183 (52.3287, 34.9463) -> (51.9834, 35.4765)
  spline S109 degree 2 poles (51.9834, 35.4765) (51.5642, 35.6984) (51.4039, 35.6984) knots 0 0 0 1 1 1
  line L184 (51.4039, 35.6984) -> (48.1858, 35.6737)
  line L185 (48.1858, 35.6737) -> (48.0748, 35.6737)
  line L186 (48.0748, 35.6737) -> (48.0748, 35.6491)
  line L187 (48.0748, 35.6491) -> (52.3533, 34.3544)
  line L188 (52.3533, 34.3544) -> (52.3533, 34.2928)
  spline S110 degree 2 poles (52.3533, 34.2928) (52.3533, 34.2188) (50.6641, 33.7379) knots 0 0 0 1 1 1
  line L189 (50.6641, 33.7379) -> (47.261, 32.7269)
  line L190 (47.261, 32.7269) -> (47.261, 32.6899)
  line L191 (47.261, 32.6899) -> (48.42, 32.6405)
  line L192 (48.42, 32.6405) -> (51.1696, 32.6405)
  line L193 (51.1696, 32.6405) -> (51.3423, 32.6899)
  line L194 (51.3423, 32.6899) -> (51.4779, 32.6652)
  spline S111 degree 2 poles (51.4779, 32.6652) (52.1807, 32.6652) (52.1807, 33.2324) knots 0 0 0 1 1 1
  spline S112 degree 2 poles (52.1807, 33.2324) (52.2917, 33.2324) (52.2917, 33.3064) knots 0 0 0 1 1 1
  line L195 (52.2917, 33.3064) -> (52.2917, 33.368)
  line L196 (52.2917, 33.368) -> (52.3533, 33.368)
  line L197 (52.3533, 33.368) -> (52.3533, 33.2817)
  line L198 (52.3533, 33.2817) -> (52.3287, 33.257)
  line L199 (52.3287, 33.257) -> (52.3533, 33.2324)
  line L200 (52.3533, 33.2324) -> (52.3533, 31.4692)
  line L201 (52.3533, 31.4692) -> (52.2917, 31.4692)
  line L202 (52.2917, 31.4692) -> (52.2917, 31.6418)
  spline S113 degree 2 poles (52.2917, 31.6418) (52.2917, 31.6788) (52.156, 31.7158) knots 0 0 0 1 1 1
  spline S114 degree 2 poles (52.156, 31.7158) (52.156, 32.1597) (51.9588, 32.1597) knots 0 0 0 1 1 1
  spline S115 degree 2 poles (51.9588, 32.1597) (51.8108, 32.2213) (51.5642, 32.2213) knots 0 0 0 1 1 1
  line L203 (51.5642, 32.2213) -> (47.2117, 32.1597)
  line L204 (47.2117, 32.1597) -> (46.7061, 32.1843)
  line L205 (46.7061, 32.1843) -> (46.6815, 32.1597)
  line L206 (46.6815, 32.1597) -> (46.6815, 32.024)
  spline S116 degree 2 poles (46.6815, 32.024) (46.6815, 31.7158) (47.187, 31.3459) knots 0 0 0 1 1 1
  line L207 (47.187, 31.3459) -> (47.8652, 30.5937)
  line L208 (47.8652, 30.5937) -> (47.8652, 30.5568)
  spline S117 degree 2 poles (47.8652, 30.5568) (47.1377, 31.1733) (46.9527, 31.1733) knots 0 0 0 1 1 1
  spline S118 degree 2 poles (46.9527, 31.1733) (46.3979, 31.6541) (46.139, 31.7528) knots 0 0 0 1 1 1
  line L209 (46.139, 31.7528) -> (46.139, 31.8021)
  line L210 (46.139, 31.8021) -> (46.2499, 31.9131)
  line L211 (46.2499, 31.9131) -> (46.1759, 32.1103)
  spline S119 degree 2 poles (46.1759, 32.1103) (46.0896, 32.1103) (46.028, 31.6911) knots 0 0 0 1 1 1
  line L212 (46.028, 31.6911) -> (45.917, 31.6911)
  line L213 (45.917, 31.6911) -> (45.8677, 31.7528)
  line L214 (45.8677, 31.7528) -> (45.8677, 32.6159)
  spline S120 degree 2 poles (45.8677, 32.6159) (45.8677, 32.7269) (45.6951, 32.9735) knots 0 0 0 1 1 1
  line L215 (49.2338, 34.0955) -> (49.2585, 34.0955)
  spline S121 degree 2 poles (49.2585, 34.0955) (49.69, 34.0955) (50.8614, 34.4654) knots 0 0 0 1 1 1
  line L216 (50.8614, 34.4654) -> (50.8614, 34.5024)
  line L217 (50.8614, 34.5024) -> (47.1007, 35.6244)
  spline S122 degree 2 poles (47.1007, 35.6244) (47.298, 35.4148) (48.3091, 34.8353) knots 0 0 0 1 1 1
  spline S123 degree 2 poles (48.3091, 34.8353) (48.8023, 34.0955) (49.2338, 34.0955) knots 0 0 0 1 1 1
  line L218 (45.7691, 40.8401) -> (45.7691, 41.3702)
  spline S124 degree 2 poles (45.7691, 41.3702) (45.7691, 42.332) (46.4842, 43.2568) knots 0 0 0 1 1 1
  spline S125 degree 2 poles (46.4842, 43.2568) (46.4842, 43.3801) (47.113, 44.2185) knots 0 0 0 1 1 1
  line L219 (47.113, 44.2185) -> (47.113, 44.1938)
  line L220 (47.113, 44.1938) -> (46.9281, 43.3307)
  line L221 (46.9281, 43.3307) -> (46.9527, 43.2937)
  line L222 (46.9527, 43.2937) -> (46.9774, 43.2937)
  spline S126 degree 2 poles (46.9774, 43.2937) (47.8035, 44.0089) (48.9009, 44.0089) knots 0 0 0 1 1 1
  line L223 (48.9009, 44.0089) -> (49.2461, 44.0089)
  spline S127 degree 2 poles (49.2461, 44.0089) (51.0587, 44.0089) (52.0697, 42.2457) knots 0 0 0 1 1 1
  spline S128 degree 2 poles (52.0697, 42.2457) (52.1684, 41.8511) (52.4643, 41.7155) knots 0 0 0 1 1 1
  spline S129 degree 2 poles (52.4643, 41.7155) (53.1055, 41.1236) (53.5124, 41.1236) knots 0 0 0 1 1 1
  spline S130 degree 2 poles (53.5124, 41.1236) (53.5493, 41.0743) (54.3878, 40.9387) knots 0 0 0 1 1 1
  line L224 (54.3878, 40.9387) -> (54.3878, 40.877)
  spline S131 degree 2 poles (54.3878, 40.877) (53.2164, 40.877) (52.193, 40.0139) knots 0 0 0 1 1 1
  spline S132 degree 2 poles (52.193, 40.0139) (51.4039, 38.0165) (49.0859, 37.9795) knots 0 0 0 1 1 1
  spline S133 degree 2 poles (49.0859, 37.9795) (47.8282, 37.9795) (46.9527, 38.7069) knots 0 0 0 1 1 1
  line L225 (46.9527, 38.7069) -> (46.9281, 38.3987)
  line L226 (46.9281, 38.3987) -> (46.9774, 37.7452)
  line L227 (46.9774, 37.7452) -> (46.9281, 37.7452)
  spline S134 degree 2 poles (46.9281, 37.7452) (45.7691, 40.0509) (45.7691, 40.8401) knots 0 0 0 1 1 1
  line L228 (48.3091, 39.8536) -> (48.5063, 39.8536)
  spline S135 degree 2 poles (48.5063, 39.8536) (50.886, 39.8536) (51.9094, 40.4085) knots 0 0 0 1 1 1
  line L229 (51.9094, 40.4085) -> (51.9711, 40.8401)
  line L230 (51.9711, 40.8401) -> (51.9711, 41.1483)
  spline S136 degree 2 poles (51.9711, 41.1483) (51.9711, 41.7525) (51.5642, 41.7525) knots 0 0 0 1 1 1
  spline S137 degree 2 poles (51.5642, 41.7525) (50.5161, 42.147) (48.5063, 42.147) knots 0 0 0 1 1 1
  spline S138 degree 2 poles (48.5063, 42.147) (46.7185, 42.147) (46.2746, 41.4072) knots 0 0 0 1 1 1
  line L231 (46.2746, 41.4072) -> (46.2376, 41.2223)
  line L232 (46.2376, 41.2223) -> (46.2376, 40.7537)
  spline S139 degree 2 poles (46.2376, 40.7537) (46.2376, 40.3592) (46.8911, 40.0386) knots 0 0 0 1 1 1
  spline S140 degree 2 poles (46.8911, 40.0386) (47.4459, 39.8536) (48.3091, 39.8536) knots 0 0 0 1 1 1
  line L233 (52.3163, 40.5688) -> (52.341, 40.5688)
  spline S141 degree 2 poles (52.341, 40.5688) (52.7232, 40.7661) (52.7972, 40.914) knots 0 0 0 1 1 1
  line L234 (52.7972, 40.914) -> (52.7972, 40.9757)
  spline S142 degree 2 poles (52.7972, 40.9757) (52.489, 41.3333) (52.3163, 41.4072) knots 0 0 0 1 1 1
  line L235 (52.3163, 41.4072) -> (52.341, 41.099)
  line L236 (52.341, 41.099) -> (52.341, 40.7907)
  line L237 (52.341, 40.7907) -> (52.3163, 40.5688)
  line L238 (49.3448, 39.0522) -> (49.5174, 39.0522)
  spline S143 degree 2 poles (49.5174, 39.0522) (50.4545, 39.0522) (51.2683, 39.607) knots 0 0 0 1 1 1
  line L239 (51.2683, 39.607) -> (51.2313, 39.607)
  spline S144 degree 2 poles (51.2313, 39.607) (49.616, 39.0892) (49.3448, 39.0892) knots 0 0 0 1 1 1
  line L240 (49.3448, 39.0892) -> (49.3448, 39.0522)
  spline S145 degree 2 poles (49.7024, 42.8869) (50.7381, 42.6156) (51.3546, 42.332) knots 0 0 0 1 1 1
  line L241 (51.3546, 42.332) -> (51.3793, 42.332)
  line L242 (51.3793, 42.332) -> (51.3793, 42.369)
  spline S146 degree 2 poles (51.3793, 42.369) (50.5778, 42.9238) (49.7763, 42.9238) knots 0 0 0 1 1 1
  line L243 (49.7763, 42.9238) -> (49.7024, 42.9238)
  line L244 (49.7024, 42.9238) -> (49.7024, 42.8869)
  point P0 (2.54, 115.6589)
  point P1 (44.1908, 6.7843)
  constraints: 1 other
extrude "Extrusion14" add sketch "Sketch15" along normal blind 1.27 contours S0 S1 L0 S2 L1 L2 S3 S4 S5 L3 S6 L4 L5 L6 S7 S8 S9 S10 S11 L7 S12 S13 L8 L9 S14 L10 L11 L12 L13 S15 S16 L14 L15 S17 L16 L17 L18 S18 L19 L20 L21 L22 S19 S20 S21 S22 L23 S23 | L32 S37 L90 L89 L88 S70 S38 L34 L35 S39 S40 L36 S41 S42 L37 L38 L39 S43 L40 S44 S45 S46 S47 S48 L41 S49 L42 S50 S51 L43 L44 L45 L46 S52 L47 L48 L49 S53 S54 S55 S56 L50 S57 L51 L52 S58 S59 L53 L54 L55 S60 L56 | L90 L91 S71 S72 S73 L92 L93 S74 L94 L95 S75 L96 L97 L98 S61 L57 L58 L59 S62 L60 L61 S89 S88 S63 L64 S64 L65 L66 L67 L68 S65 L69 L70 L71 L72 S66 L73 L74 L75 L76 L77 L78 L79 L80 L81 S67 L82 S68 L83 L84 S69 L85 L86 L87 S70 S38 L33 S37 | S37 L33 S38 S70 L88 L89 L90 | S89 S90 L143 S91 S92 L144 S93 S94 L108 L109 L110 L111 L112 L113 L114 L115 S77 S118 S78 S79 L118 S117 L208 L207 S80 L119 S81 L120 L121 L122 S82 L123 L124 L125 S83 S84 L126 L127 L128 S85 L129 L130 L131 L132 L133 L134 L135 S86 S87 L136 L137 L138 L139 L140 L141 L61 | L61 L141 S63 S88 S89 | L61 L62 L63 S63 L141 | L141 L142 S88 S63 | S118 L209 L210 L211 S119 L212 L213 L214 S120 L169 S104 L170 S105 L171 L172 L173 L174 L175 L176 S106 S107 L177 L178 L179 S108 L180 L181 L182 L183 S109 L184 L185 L186 L187 L188 S110 L189 L190 L191 L192 L193 L194 S111 S112 L195 L196 L197 L198 L199 L200 L201 L202 S113 S114 S115 L203 L204 L205 L206 S116 L207 L118 S117 S78 L117 L116 S77 | S77 L116 L117 S78 S118 | L118 L207 L208 S117 | L218 S124 S125 L219 L220 L221 L222 S126 L223 S127 S128 S129 S130 L224 S131 S132 S133 L225 L226 L227 S134
body "Solid1"
